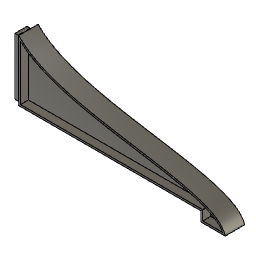
christmas-tree-stand (Autodesk Fusion 360 design; units mm, degrees)
Autodesk Fusion 360 part; units mm, degrees
sketch "Sketch1" plane through (0, 0, 0) normal (0, 1, 0) x (1, 0, 0)
  line L0 (0, 0) -> (170, 0)
  line L1 (170, 0) -> (170, -58)
  line L2 (170, -58) -> (0, -58)
  line L3 (0, -58) -> (0, 0)
  line L4 (0, 0) -> (150, 0)
  line L5 (150, 0) -> (150, -8)
  line L6 (150, -8) -> (0, -8)
  line L7 (0, -8) -> (0, 0)
  spline S0 degree 5 poles (0, -58) (1.1045, -56.8163) (3.5, -54.4999) (7.6532, -51.178) (14.3184, -47.0563) (24.5496, -42.4239) (36.6533, -38.3087) (50.505, -34.6869) (65.8217, -31.4981) (82.1025, -28.6313) (98.7056, -25.943) (114.9146, -23.2722) (130.0015, -20.4555) (143.2957, -17.342) (154.2452, -13.8074) (162.5118, -9.7738) (166.8955, -6.127) (168.931, -3.1549) (169.7357, -1.0691) (170, 0) knots 0 0 0 0 0 0 0.066667 0.133333 0.2 0.266667 0.333333 0.4 0.466667 0.533333 0.6 0.666667 0.733333 0.8 0.866667 0.933333 1 1 1 1 1 1
  point P0 (50, -35)
  point P1 (150, -15)
  dimension "d1" = 170
  dimension "d2" = 58
  dimension "d3" = 150
  dimension "d4" = 8
  constraint horizontal L0
  constraint vertical L1
  constraint horizontal L2
  constraint vertical L3
  constraint coincident L0.start L3.end
  constraint horizontal L4
  constraint vertical L5
  constraint horizontal L6
  constraint vertical L7
  measures "d1" distance of L0.start L0.end
  measures "d2" distance of L0.start L2.end
  measures "d3" distance of L0.start L4.end
  measures "d4" distance of L0.start L6.end
extrude "Extrude1" add sketch "Sketch1" along normal blind 8 contours L0 L3 L5 L6 S0 makes body 1
shell "Shell1" thickness 1.5 removed faces 1 at (61.3506, 8, 20.8158) on bodies 1
sketch "Sketch2" plane through (0, 0, 0) normal (0, 1, 0) x (1, 0, 0)
  line L0 (0, -8) -> (-3.5, -8)
  line L1 (-3.5, -8) -> (-3.5, -55)
  line L2 (-3.5, -55) -> (0, -55)
  line L3 (0, -55) -> (0, -8)
  dimension "d8" = 3.5
  dimension "d9" = 47
  constraint horizontal L0
  constraint vertical L1
  constraint horizontal L2
  constraint vertical L3
  measures "d8" distance of L0.start L0.end
  measures "d9" distance of L0.start L2.end
extrude "Extrude2" add sketch "Sketch2" along normal blind 1.75 bodies 1
sketch "Sketch3" plane through (0, 0, 0) normal (0, 1, 0) x (1, 0, 0)
  line L0 (-3.5, -55) -> (-6.1, -55)
  line L1 (-6.1, -55) -> (-6.1, -8)
  line L2 (-6.1, -8) -> (-3.5, -8)
  line L3 (-3.5, -8) -> (-3.5, -55)
  point P0 (-3.5, -55)
  dimension "d12" = 2.6
  dimension "d13" = 47
  constraint horizontal L0
  constraint vertical L1
  constraint horizontal L2
  constraint vertical L3
  constraint coincident P0 L0.start
  measures "d12" distance of P0 L0.end
  measures "d13" distance of P0 L2.end
extrude "Extrude3" add sketch "Sketch3" along normal blind 5 bodies 1
copy_body "Body->Comp1" bodies 1 removing the originals makes body 2 in component "Component"
mirror "Mirror1" about plane through (0, 0, 0) normal (0, 1, 0) of bodies 2 merged in component "Component"
component "Component" placed x (1, 0, 0) y (0, 1, 0) z (0, 0, 1) at (0, 0, 0)
